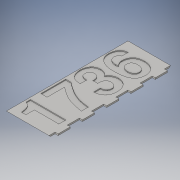
# Autodesk Inventor part: side
Saved by Autodesk Inventor 2016 (Build 200138000, 138)
## iProperties
Created: 2015-08-25
Part Number: side
Material: Generic
Document SubType Name: Modeling
Designer: gerthcm
Density: 1 g/cm^3
Appearance: Default
Author: gerthcm
Autodesk Inventor part; units mm, degrees
ref_plane "YZ Plane" through (0, 0, 0) normal (1, 0, 0) x (0, 1, 0)
ref_plane "XZ Plane" through (0, 0, 0) normal (0, 1, 0) x (-1, 0, 0)
ref_plane "XY Plane" through (0, 0, 0) normal (0, 0, 1) x (1, 0, 0)
sketch "Sketch1" plane through (0, 0, 0) normal (0, 1, 0) x (-1, 0, 0)
  line L0 (44.45, 127) -> (-44.45, 127)
  line L1 (-44.45, 127) -> (-44.45, -127)
  line L2 (-44.45, -127) -> (44.45, -127)
  line L3 (44.45, -127) -> (44.45, 127)
  point P0 (0, 0)
  dimension "d0" = 88.9
  dimension "d1" = 254
  constraints: 8 end point, 2 parallel, 1 horizontal, 1 perpendicular
  measures "d0" distance of L2.end L1.end
  measures "d1" distance of L1.end L0.end
extrude "Extrusion1" add sketch "Sketch1" along normal blind 3.175
sketch "Sketch3" plane through (0, 3.175, 0) normal (0, 1, 0) x (1, 0, 0)
  line L0 (50.8, -114.3) -> (44.45, -114.3)
  line L1 (44.45, -114.3) -> (44.45, -88.9)
  line L2 (44.45, -88.9) -> (50.8, -88.9)
  line L3 (50.8, -88.9) -> (50.8, -114.3)
  line L4 (50.8, -63.5) -> (44.45, -63.5)
  line L5 (44.45, -63.5) -> (44.45, -38.1)
  line L6 (44.45, -38.1) -> (50.8, -38.1)
  line L7 (50.8, -38.1) -> (50.8, -63.5)
  line L8 (50.8, -12.7) -> (44.45, -12.7)
  line L9 (44.45, -12.7) -> (44.45, 12.7)
  line L10 (44.45, 12.7) -> (50.8, 12.7)
  line L11 (50.8, 12.7) -> (50.8, -12.7)
  line L12 (50.8, 38.1) -> (44.45, 38.1)
  line L13 (44.45, 38.1) -> (44.45, 63.5)
  line L14 (44.45, 63.5) -> (50.8, 63.5)
  line L15 (50.8, 63.5) -> (50.8, 38.1)
  line L16 (50.8, 88.9) -> (44.45, 88.9)
  line L17 (44.45, 88.9) -> (44.45, 114.3)
  line L18 (44.45, 114.3) -> (50.8, 114.3)
  line L19 (50.8, 114.3) -> (50.8, 88.9)
  point P0 (0, 0)
  dimension "d6" = 50.8
  constraints: 40 end point, 2 parallel, 1 collinear, 1 horizontal, 1 perpendicular, 1 vertical, 31 other
  measures "d6" distance of L0.start L4.start
extrude "Extrusion2" add sketch "Sketch3" against normal blind 3.175
sketch "Sketch4" plane through (44.042, 3.175, 128.8813) normal (0, 1, 0) x (0, 0, -1)
  line L0 (8.2401, 85.8951) -> (239.8135, 85.8951) construction
  line L1 (239.8135, 85.8951) -> (239.8135, 3.5919) construction
  line L2 (239.8135, 3.5919) -> (8.2401, 3.5919) construction
  line L3 (8.2401, 3.5919) -> (8.2401, 85.8951) construction
  line L4 (47.8214, 10.1099) -> (33.1858, 10.1099)
  line L5 (33.1858, 10.1099) -> (33.1858, 61.3049)
  line L6 (33.1858, 61.3049) -> (15.4097, 61.3049)
  line L7 (15.4097, 61.3049) -> (15.4097, 70.8447)
  spline S0 degree 2 poles (15.4097, 70.8447) (25.9569, 71.9112) (30.4601, 74.2221) knots 0 0 0 1 1 1
  spline S1 degree 2 poles (30.4601, 74.2221) (35.6744, 77.007) (38.5186, 84.236) knots 0 0 0 1 1 1
  line L8 (38.5186, 84.236) -> (47.8214, 84.236)
  line L9 (47.8214, 84.236) -> (47.8214, 10.1099)
  spline S2 degree 2 poles (121.5327, 73.0371) (102.9271, 49.8689) (98.0091, 30.1968) knots 0 0 0 1 1 1
  spline S3 degree 2 poles (98.0091, 30.1968) (96.0537, 22.2568) (94.8687, 10.1099) knots 0 0 0 1 1 1
  line L10 (94.8687, 10.1099) -> (79.9368, 10.1099)
  spline S4 degree 2 poles (79.9368, 10.1099) (83.7883, 33.1002) (93.0911, 54.1352) (105.9491, 71.0817) knots 0 0 0 1 2 2 2
  line L11 (105.9491, 71.0817) -> (69.3897, 71.0817)
  line L12 (69.3897, 71.0817) -> (69.3897, 84.236)
  line L13 (69.3897, 84.236) -> (121.5327, 84.236)
  line L14 (121.5327, 84.236) -> (121.5327, 73.0371)
  spline S5 degree 2 poles (178.5939, 31.3226) (178.5939, 20.4792) (164.373, 7.6212) (152.4631, 7.6212) knots 0 0 0 1 2 2 2
  spline S6 degree 2 poles (152.4631, 7.6212) (142.5085, 7.6212) (135.8128, 12.8355) knots 0 0 0 1 1 1
  spline S7 degree 2 poles (135.8128, 12.8355) (127.5766, 19.2941) (127.5766, 31.8559) knots 0 0 0 1 1 1
  line L15 (127.5766, 31.8559) -> (141.7974, 31.8559)
  spline S8 degree 2 poles (141.7974, 31.8559) (141.2642, 25.3973) (145.5897, 21.9605) knots 0 0 0 1 1 1
  spline S9 degree 2 poles (145.5897, 21.9605) (148.9079, 19.2349) (153.7074, 19.2349) knots 0 0 0 1 1 1
  spline S10 degree 2 poles (153.7074, 19.2349) (157.6181, 19.2349) (163.7805, 27.2934) (163.7805, 31.7966) knots 0 0 0 1 2 2 2
  spline S11 degree 2 poles (163.7805, 31.7966) (163.7805, 37.485) (154.8925, 43.7066) (147.2488, 43.3511) knots 0 0 0 1 2 2 2
  line L16 (147.2488, 43.3511) -> (147.2488, 53.3057)
  spline S12 degree 2 poles (147.2488, 53.3057) (162.0621, 52.8909) (162.0621, 64.5638) knots 0 0 0 1 1 1
  spline S13 degree 2 poles (162.0621, 64.5638) (162.0621, 74.2814) (151.8113, 74.2814) knots 0 0 0 1 1 1
  spline S14 degree 2 poles (151.8113, 74.2814) (147.2488, 74.2814) (145.1156, 71.9705) knots 0 0 0 1 1 1
  spline S15 degree 2 poles (145.1156, 71.9705) (142.39, 68.9486) (142.0937, 60.8901) knots 0 0 0 1 1 1
  line L17 (142.0937, 60.8901) -> (128.7024, 60.8901)
  spline S16 degree 2 poles (128.7024, 60.8901) (128.5247, 62.5492) (128.5247, 64.149) knots 0 0 0 1 1 1
  spline S17 degree 2 poles (128.5247, 64.149) (128.5247, 73.7481) (142.2122, 85.8951) (152.6408, 85.8951) knots 0 0 0 1 2 2 2
  spline S18 degree 2 poles (152.6408, 85.8951) (163.1287, 85.8951) (169.3503, 80.977) knots 0 0 0 1 1 1
  spline S19 degree 2 poles (169.3503, 80.977) (176.1645, 75.7627) (176.1645, 66.0452) knots 0 0 0 1 1 1
  spline S20 degree 2 poles (176.1645, 66.0452) (176.1645, 60.4161) (174.2684, 56.9201) knots 0 0 0 1 1 1
  spline S21 degree 2 poles (174.2684, 56.9201) (172.7278, 54.2537) (168.0467, 49.8689) knots 0 0 0 1 1 1
  spline S22 degree 2 poles (168.0467, 49.8689) (178.5939, 43.0548) (178.5939, 31.3226) knots 0 0 0 1 1 1
  spline S23 degree 2 poles (236.7808, 34.7001) (236.7808, 22.8494) (230.0852, 15.3242) knots 0 0 0 1 1 1
  spline S24 degree 2 poles (230.0852, 15.3242) (223.0932, 7.6212) (211.4796, 7.6212) knots 0 0 0 1 1 1
  spline S25 degree 2 poles (211.4796, 7.6212) (195.4811, 7.6212) (189.7335, 22.4346) knots 0 0 0 1 1 1
  spline S26 degree 2 poles (189.7335, 22.4346) (186.0006, 32.0929) (186.0006, 51.4095) knots 0 0 0 1 1 1
  spline S27 degree 2 poles (186.0006, 51.4095) (186.0006, 66.2229) (192.874, 75.7627) knots 0 0 0 1 1 1
  spline S28 degree 2 poles (192.874, 75.7627) (200.2214, 85.8951) (212.7831, 85.8951) knots 0 0 0 1 1 1
  spline S29 degree 2 poles (212.7831, 85.8951) (222.56, 85.8951) (234.9439, 75.9997) (235.5365, 67.408) knots 0 0 0 1 2 2 2
  line L18 (235.5365, 67.408) -> (222.0859, 67.408)
  spline S30 degree 2 poles (222.0859, 67.408) (219.538, 74.1629) (212.1313, 74.1629) knots 0 0 0 1 1 1
  spline S31 degree 2 poles (212.1313, 74.1629) (206.7985, 74.1629) (200.2214, 65.5119) (200.2214, 58.52) knots 0 0 0 1 2 2 2
  spline S32 degree 2 poles (200.2214, 58.52) (200.2214, 56.0906) (200.6362, 53.4834) knots 0 0 0 1 1 1
  spline S33 degree 2 poles (200.6362, 53.4834) (207.3318, 59.231) (213.4942, 59.231) knots 0 0 0 1 1 1
  spline S34 degree 2 poles (213.4942, 59.231) (224.3376, 59.231) (236.7808, 46.6693) (236.7808, 34.7001) knots 0 0 0 1 2 2 2
  spline S35 degree 2 poles (222.9747, 35.1148) (222.9747, 41.1587) (217.2864, 47.8543) (212.3091, 47.8543) knots 0 0 0 1 2 2 2
  spline S36 degree 2 poles (212.3091, 47.8543) (207.1541, 47.8543) (200.2214, 39.7959) (200.2214, 33.1002) knots 0 0 0 1 2 2 2
  spline S37 degree 2 poles (200.2214, 33.1002) (200.2214, 27.5896) (206.5023, 19.9459) (211.1833, 19.9459) knots 0 0 0 1 2 2 2
  spline S38 degree 2 poles (211.1833, 19.9459) (216.5754, 19.9459) (222.9747, 28.3007) (222.9747, 35.1148) knots 0 0 0 1 2 2 2
  point P0 (127, 0)
  constraints: 2 other
extrude "Extrusion3" cut sketch "Sketch4" against normal blind 1.905
chamfer "Chamfer1" distance 3.175 angle 45 2 edges at (0, 0, 127) (0, 0, -127)
body "Solid1"
